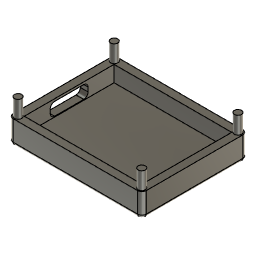
_part 2.af4cea7a-fd4b-4f0e-be85-1c45aad45d52 (Autodesk Fusion 360 design; units mm, degrees)
Autodesk Fusion 360 part; units mm, degrees
sketch "Sketch1" plane through (0, 0, 0) normal (0, 0, 1) x (1, 0, 0)
  line L0 (-15.5, 12.25) -> (15.5, 12.25)
  line L1 (15.5, 12.25) -> (15.5, -12.25)
  line L2 (15.5, -12.25) -> (-15.5, -12.25)
  line L3 (-15.5, -12.25) -> (-15.5, 12.25)
  line L4 (-15.5, 12.25) -> (15.5, -12.25) construction
  line L5 (15.5, 12.25) -> (-15.5, -12.25) construction
  dimension "d1" = 31
  dimension "d2" = 24.5
  constraint horizontal L0
  constraint perpendicular L0 L1
  constraint parallel L0 L2
  constraint parallel L1 L3
  constraint coincident L4 origin
  constraint coincident L5 origin
  measures "d1" distance of L0.start L0.end
  measures "d2" distance of L0.start L2.end
extrude "Extrude1" add sketch "Sketch1" along normal blind 5.5
shell "Shell1" thickness 1.8 removed faces 1 at (-5.1667, 4.0833, 5.5)
sketch "Sketch2" plane through (0, 0, 5.5) normal (0, 0, 1) x (-1, 0, 0)
  line L0 (13.7, 10.45) -> (13.7, -10.45)
  line L1 (13.7, -10.45) -> (-13.7, -10.45)
  line L2 (-13.7, -10.45) -> (-13.7, 10.45)
  line L3 (-13.7, 10.45) -> (13.7, 10.45)
  line L4 (15.5, 12.25) -> (-15.5, 12.25)
  line L5 (-15.5, 12.25) -> (-15.5, -12.25)
  line L6 (-15.5, -12.25) -> (15.5, -12.25)
  line L7 (15.5, -12.25) -> (15.5, 12.25)
  circle A0 centre (14.4, -11.2) radius 0.84
  line L8 (0, 0) -> (0, -2)
  line L9 (0, 0) -> (4, 0)
  circle A1 centre (-14.4, -11.2) radius 0.84
  circle A2 centre (-14.4, 11.2) radius 0.84
  circle A3 centre (14.4, 11.2) radius 0.84
  dimension "d6" = 1.68
  dimension "d7" = 11.2
  dimension "d8" = 14.4
  constraint coincident L8.start L9.start
  constraint vertical L8
  constraint perpendicular L8 L9
  constraint symmetric A0 L8 A1
  constraint symmetric A0 L9 A3
  constraint symmetric L9 A1 A2
  measures "d6" diameter of A0
  measures "d7" vertical distance of L8.start A0.centre
  measures "d8" horizontal distance of L8.start A0.centre
extrude "Extrude2" add sketch "Sketch2" along normal blind 4 contours A0 | A1 | A2 | A3
fillet "Fillet1" radius 1 1 edges at (15.5, -12.25, 2.75)
fillet "Fillet1" radius 1 1 edges at (15.5, 12.25, 2.75)
fillet "Fillet1" radius 1 1 edges at (-15.5, 12.25, 2.75)
fillet "Fillet1" radius 1 1 edges at (-15.5, -12.25, 2.75)
sketch "Sketch3" plane through (-15.5, 0, 0) normal (-1, 0, 0) x (0, -1, 0)
  line L0 (11.25, 0) -> (11.25, 5.5)
  line L1 (11.25, 5.5) -> (-11.25, 5.5)
  line L2 (-11.25, 5.5) -> (-11.25, 0)
  line L3 (-11.25, 0) -> (11.25, 0)
  line L4 (0, 0) -> (0, 1.96)
  line L5 (0, 1.96) -> (0, 3.46)
  line L6 (-3.4, 1.96) -> (3.4, 1.96)
  line L7 (4.4, 2.96) -> (4.4, 3.96)
  line L8 (3.4, 4.96) -> (-3.4, 4.96)
  line L9 (-4.4, 3.96) -> (-4.4, 2.96)
  line L10 (-4.4, 1.96) -> (4.4, 4.96) construction
  line L11 (4.4, 1.96) -> (-4.4, 4.96) construction
  arc A0 (-3.4, 4.96) -> (-4.4, 3.96) centre (-3.4, 3.96) ccw
  arc A1 (-4.4, 2.96) -> (-3.4, 1.96) centre (-3.4, 2.96) ccw
  arc A2 (3.4, 1.96) -> (4.4, 2.96) centre (3.4, 2.96) ccw
  arc A3 (4.4, 3.96) -> (3.4, 4.96) centre (3.4, 3.96) ccw
  point P0 (0, 3.46)
  dimension "d19" = 1.96
  dimension "d20" = 1.5
  dimension "d21" = 3
  dimension "d22" = 8.8
  dimension "d23" = 1
  constraint coincident L4.start origin
  constraint perpendicular L3 L4
  constraint parallel L4 L5
  constraint horizontal L6
  constraint perpendicular L6 L7
  constraint parallel L6 L8
  constraint parallel L7 L9
  constraint coincident L10 P0
  constraint coincident L11 P0
  constraint coincident P0 L5.end
  constraint coincident L11.end L9
  constraint coincident L11.end L8
  constraint tangent L9 A0
  constraint tangent L8 A0
  constraint coincident L10.start L9
  constraint coincident L10.start L6
  constraint tangent L9 A1
  constraint tangent L6 A1
  constraint equal A0 A1
  constraint coincident L11.start L6
  constraint coincident L11.start L7
  constraint tangent L6 A2
  constraint tangent L7 A2
  constraint equal A0 A2
  constraint coincident L10.end L7
  constraint coincident L10.end L8
  constraint tangent L7 A3
  constraint tangent L8 A3
  constraint equal A0 A3
  measures "d19" distance of L4.start L4.end
  measures "d20" distance of L4.end P0
  measures "d21" distance of L10.start L11.end
  measures "d22" distance of L10.end L11.end
  measures "d23" radius of A0
extrude "Extrude3" cut sketch "Sketch3" against normal blind 6 contours L6 L7 L8 L9 A0 A1 A2 A3
fillet "Fillet2" radius 0.75 8 edges at (-15.2071, -11.9571, 0) (-15.5, 0, 0) (-15.2071, 11.9571, 0) (0, 12.25, 0) (15.2071, 11.9571, 0) (15.5, 0, 0) (15.2071, -11.9571, 0) (0, -12.25, 0)
